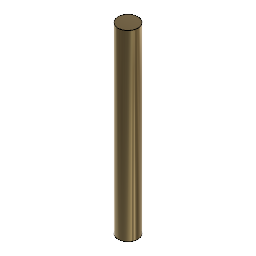
Union v2 (Autodesk Fusion 360 design; units mm, degrees)
Autodesk Fusion 360 part; units mm, degrees
sketch "Boceto2" plane through (0, 0, 0) normal (0, 0, 1) x (1, 0, 0)
  circle A0 centre (0, 0) radius 5.5
  dimension "d5" = 11
  constraint coincident A0.centre origin
  measures "d5" diameter of A0
extrude "Extruir2" add sketch "Boceto2" along normal mid plane 100
